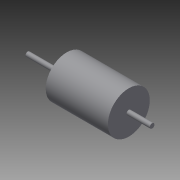
# Autodesk Inventor part: Rotor
Saved by Autodesk Inventor 2015 (Build 190159000, 159)
## iProperties
Created: 2014-08-26
Part Number: Rotor
Material: Generic
Document SubType Name: Modeling
Designer: laca
Density: 1 g/cm^3
Appearance: Default
Mass: 23.185 g
Surface Area: 49.1502 cm^2
Volume: 23.185 cm^3
Author: laca
Autodesk Inventor part; units mm, degrees
ref_plane "YZ Plane" through (0, 0, 0) normal (1, 0, 0) x (0, 1, 0)
ref_plane "XZ Plane" through (0, 0, 0) normal (0, 1, 0) x (-1, 0, 0)
ref_plane "XY Plane" through (0, 0, 0) normal (0, 0, 1) x (1, 0, 0)
sketch "Sketch1" plane through (0, 0, 0) normal (0, 0, 1) x (1, 0, 0)
  line L0 (-60.9516, 17.35) -> (-35.9516, 17.35)
  line L1 (-35.9516, 17.35) -> (-35.9516, 29.35)
  line L2 (-35.9516, 29.35) -> (4.0484, 29.35)
  line L3 (4.0484, 29.35) -> (4.0484, 17.35)
  line L4 (4.0484, 17.35) -> (19.0484, 17.35)
  line L5 (19.0484, 17.35) -> (19.0484, 15.85)
  line L6 (19.0484, 15.85) -> (-60.9516, 15.85)
  line L7 (-60.9516, 15.85) -> (-60.9516, 17.35)
  point P0 (0, 0)
  dimension "d2" = 1.5
  dimension "d3" = 12
  dimension "d4" = 40
  dimension "d5" = 15
  dimension "d6" = 25
  constraints: 16 end point, 6 perpendicular, 2 point on line, 1 horizontal
  measures "d2" distance of L6.end L0.start
  measures "d3" distance of L0.end L1.end
  measures "d4" distance of L1.end L2.end
  measures "d5" distance of L3.end L4.end
  measures "d6" distance of L0.start L0.end
revolve "Revolution1" add sketch "Sketch1" angle 360 about axis through (19.0484, 15.85, 0) along (-1, 0, 0)
body "Solid1"
